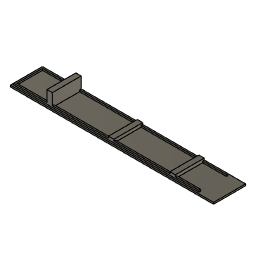
Case_moisture_sensor v6 (Autodesk Fusion 360 archive; units mm, degrees)
design "Lid_moisture_sensor"
Autodesk Fusion 360 part; units mm, degrees
sketch "Sketch1" plane through (0, 0, 0) normal (0, 0, 1) x (1, 0, 0)
  line L0 (0, 0) -> (190, 0)
  line L1 (190, 0) -> (190, 30)
  line L2 (190, 30) -> (0, 30)
  line L3 (0, 30) -> (0, 0)
  dimension "d1" = 190
  dimension "d2" = 30
  constraint horizontal L0
  constraint vertical L1
  constraint horizontal L2
  constraint vertical L3
  constraint coincident L0.start L3.end
  measures "d1" distance of L0.start L0.end
  measures "d2" distance of L0.start L2.end
extrude "Extrude1" add sketch "Sketch1" along normal blind 1.5
sketch "Sketch2" plane through (0, 0, 1.5) normal (0, 0, 1) x (-1, 0, 0)
  line L0 (0, -30) -> (0, 0)
  line L1 (0, 0) -> (-190, 0)
  line L2 (-190, 0) -> (-190, -30)
  line L3 (-190, -30) -> (0, -30)
  line L4 (-1.5, -1.5) -> (-188.5, -1.5)
  line L5 (-188.5, -1.5) -> (-188.5, -28.5)
  line L6 (-188.5, -28.5) -> (-1.5, -28.5)
  line L7 (-1.5, -28.5) -> (-1.5, -1.5)
  line L8 (-32.75, -28.5) -> (-37.75, -28.5)
  line L9 (-37.75, -28.5) -> (-37.75, -1.5)
  line L10 (-37.75, -1.5) -> (-32.75, -1.5)
  line L11 (-32.75, -1.5) -> (-32.75, -28.5)
  line L12 (-188.5, -28.5) -> (-157.25, -28.5)
  line L13 (-90.25, -28.5) -> (-95.25, -28.5)
  line L14 (-90.25, -1.5) -> (-90.25, -28.5)
  line L15 (-95.25, -28.5) -> (-95.25, -1.5)
  line L16 (-95.25, -1.5) -> (-90.25, -1.5)
  line L17 (-147.75, -28.5) -> (-152.75, -28.5)
  line L18 (-147.75, -1.5) -> (-147.75, -28.5)
  line L19 (-152.75, -28.5) -> (-152.75, -1.5)
  line L20 (-152.75, -1.5) -> (-147.75, -1.5)
  dimension "d5" = -1.5
  dimension "d6" = 5
  dimension "d7" = 31.25
  dimension "d8" = 31.25
  dimension "d11" = -115
  dimension "d12" = 0
  constraint horizontal L8
  constraint vertical L9
  constraint horizontal L10
  constraint vertical L11
  constraint coincident L4 L9.end
  constraint coincident L6 L8.start
  constraint perpendicular L5 L12
  measures "d6" distance of L8.start L8.end
  measures "d7" distance of L7 L11
  measures "d8" distance of L5.end L12.end
extrude "Extrude2" add sketch "Sketch2" along normal blind 12 contours L4 L6 L8 L9 L10 L11
extrude "Extrude3" add sketch "Sketch2" along normal blind 3 contours L4 L6 L13 L14 L15 L16 | L4 L6 L17 L18 L19 L20
extrude "Extrude4" add sketch "Sketch2" along normal blind 1.5 contours L4 L6 L7 L11
sketch "Sketch3" plane through (0, 0, 3) normal (0, 0, 1) x (-1, 0, 0)
  line L0 (-32.75, -1.5) -> (-32.75, -28.5)
  line L1 (-32.75, -28.5) -> (-1.5, -28.5)
  line L2 (-1.5, -28.5) -> (-1.5, -1.5)
  line L3 (-1.5, -1.5) -> (-32.75, -1.5)
  line L4 (-3, -3) -> (-31.25, -3)
  line L5 (-31.25, -27) -> (-3, -27)
  line L6 (-3, -27) -> (-3, -3)
  line L7 (-31.25, -3) -> (-32.75, -3)
  line L8 (-31.25, -27) -> (-32.75, -27)
  constraint parallel L3 L4
  constraint parallel L1 L5
  constraint parallel L2 L6
  constraint coincident L0 L7.end
  constraint perpendicular L0 L7
  constraint coincident L0 L8.end
  constraint perpendicular L0 L8
extrude "Extrude5" cut sketch "Sketch3" against normal blind 1.5 contours L0 L4 L5 L6 L7 L8
sketch "Sketch4" plane through (0, 0, 1.5) normal (0, 0, 1) x (-1, 0, 0)
  line L0 (0, -30) -> (0, 0)
  line L1 (0, 0) -> (-190, 0)
  line L2 (-190, 0) -> (-190, -30)
  line L3 (-190, -30) -> (0, -30)
  line L4 (-37.75, -1.5) -> (-1.5, -1.5)
  line L5 (-1.5, -1.5) -> (-1.5, -28.5)
  line L6 (-1.5, -28.5) -> (-37.75, -28.5)
  line L7 (-37.75, -28.5) -> (-37.75, -1.5)
  line L8 (-95.25, -1.5) -> (-90.25, -1.5)
  line L9 (-90.25, -1.5) -> (-90.25, -28.5)
  line L10 (-90.25, -28.5) -> (-95.25, -28.5)
  line L11 (-95.25, -28.5) -> (-95.25, -1.5)
  line L12 (-152.75, -1.5) -> (-147.75, -1.5)
  line L13 (-147.75, -1.5) -> (-147.75, -28.5)
  line L14 (-147.75, -28.5) -> (-152.75, -28.5)
  line L15 (-152.75, -28.5) -> (-152.75, -1.5)
  line L16 (-190, -28.5) -> (-37.75, -28.5)
  line L17 (-37.75, -28.5) -> (-37.75, -27)
  line L18 (-37.75, -27) -> (-190, -27)
  line L19 (-190, -27) -> (-190, -28.5)
  line L20 (-190, -1.5) -> (-37.75, -1.5)
  line L21 (-37.75, -1.5) -> (-37.75, -3)
  line L22 (-37.75, -3) -> (-190, -3)
  line L23 (-190, -3) -> (-190, -1.5)
  line L24 (0, 0) -> (-190, 0)
  line L25 (-190, -30) -> (0, -30)
  line L26 (-95.25, -28.5) -> (-95.25, -1.5)
  line L27 (-37.75, -28.5) -> (-37.75, -1.5)
  line L28 (-175, -28.5) -> (-175, -27)
  line L29 (-175, -3) -> (-175, -1.5)
  line L30 (-190, 0) -> (-190, -30)
  dimension "d22" = 1.5
  dimension "d23" = 1.5
  dimension "d24" = 1.5
  dimension "d25" = 1.5
  dimension "d26" = 15
  dimension "d27" = 15
  constraint horizontal L16
  constraint vertical L17
  constraint horizontal L18
  constraint vertical L19
  constraint coincident L2 L16.start
  constraint horizontal L20
  constraint vertical L21
  constraint horizontal L22
  constraint vertical L23
  constraint coincident L2 L20.start
  constraint collinear L17 L21
  constraint collinear L21 L27
  constraint coincident L16 L28.start
  constraint coincident L18 L28.end
  constraint perpendicular L18 L28
  constraint coincident L22 L29.start
  constraint coincident L20 L29.end
  constraint perpendicular L20 L29
  measures "d22" distance of L16.start L18.end
  measures "d23" distance of L20.start L22.end
  measures "d24" distance of L20 L24
  measures "d25" distance of L16 L25
  measures "d26" distance of L23 L29
  measures "d27" distance of L28 L30
extrude "Extrude6" add sketch "Sketch4" along normal blind 1.5 contours L15 L16 L18 L28 | L15 L20 L22 L29 | L11 L13 L16 L18 L26 | L11 L13 L20 L22 L26 | L7 L9 L16 L17 L18 L27 | L7 L9 L20 L21 L22 L27
component "Lid" placed x (1, 0, 0) y (0, 1, 0) z (0, 0, 1) at (0, 0, 0)
